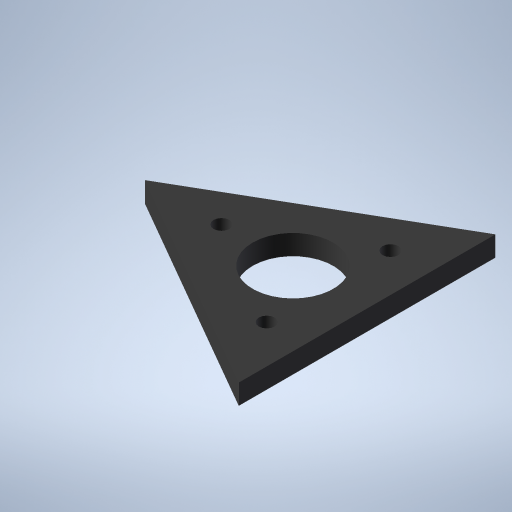
# Autodesk Inventor part: AP-1-01-planetCarrier
Saved by Autodesk Inventor 2023 (Build 270158000, 158)
## iProperties
Created: 2023-07-11
Part Number: AP-1-01-planetCarrier
Material: Generic
Document SubType Name: Modeling
Designer: t205b
Density: 1 g/cm^3
Appearance: Default
Author: t205b
Autodesk Inventor part; units mm, degrees
ref_plane "YZ Plane" through (0, 0, 0) normal (1, 0, 0) x (0, 1, 0)
ref_plane "XZ Plane" through (0, 0, 0) normal (0, 1, 0) x (-1, 0, 0)
ref_plane "XY Plane" through (0, 0, 0) normal (0, 0, 1) x (1, 0, 0)
sketch "Sketch1" plane through (0, 0, 0) normal (0, 1, 0) x (-1, 0, 0)
  line L0 (109.9852, -63.5) -> (0, 0)
  line L1 (0, 0) -> (0, -127)
  line L2 (0, -127) -> (109.9852, -63.5)
  circle A0 centre (36.6617, -63.5) radius 20
  line L3 (54.9926, -95.25) -> (46.6617, -80.8205) construction
  line L4 (54.9926, -31.75) -> (46.6617, -46.1795) construction
  line L5 (16.6617, -63.5) -> (0, -63.5) construction
  circle A1 centre (72.0735, -63.5) radius 4
  circle A2 centre (18.9559, -94.1675) radius 4
  circle A3 centre (18.9559, -32.8325) radius 4
  line L6 (18.9559, -94.1675) -> (36.6617, -63.5) construction
  line L7 (36.6617, -63.5) -> (72.0735, -63.5) construction
  line L8 (36.6617, -63.5) -> (18.9559, -32.8325) construction
  dimension "d0" = 127
  dimension "d1" = 40
  dimension "d2" = 73.3235
  dimension "d3" = 35.4117
  dimension "d4" = 8
  dimension "d5" = 120
  dimension "d6" = 120
  constraints: 18 end point, 6 equal length, 4 centre point, 3 line through centre, 3 midpoint, 3 point on circle, 2 equal radius, 2 perpendicular, 1 coincident, 1 horizontal, 1 vertical
  measures "d0" distance of L0.end L1.end
  measures "d1" diameter of A0
  measures "d2" distance of L1.end L6.end
  measures "d3" distance of L6.start L6.end
  measures "d4" diameter of A2
  measures "d5" angle of L6 L7
  measures "d6" angle of L8 L7
extrude "Extrusion1" add sketch "Sketch1" along normal blind 10
body "Solid1"
